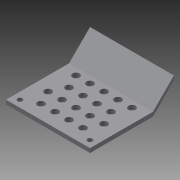
# Autodesk Inventor part: rejilla.ventilador
Saved by Autodesk Inventor 2015 SP1 (Build 190203100, 203)
## iProperties
Created: 2015-07-09
Part Number: rejilla.ventilador
Material: Generic
Document SubType Name: Modeling
Designer: pc
Density: 1 g/cm^3
Appearance: Default
Author: pc
Autodesk Inventor part; units mm, degrees
ref_plane "YZ Plane" through (0, 0, 0) normal (1, 0, 0) x (0, 1, 0)
ref_plane "XZ Plane" through (0, 0, 0) normal (0, 1, 0) x (-1, 0, 0)
ref_plane "XY Plane" through (0, 0, 0) normal (0, 0, 1) x (1, 0, 0)
sketch "Sketch3" plane through (0, 0, 0) normal (1, 0, 0) x (0, 1, 0)
  line L0 (0, 0) -> (45, 0)
  line L1 (45, 0) -> (60, 15)
  line L2 (0, 0) -> (0, 3)
  line L3 (0, 3) -> (45, 3)
  line L4 (45, 3) -> (60, 18)
  line L5 (60, 18) -> (60, 15)
  dimension "d7" = 45
  dimension "d8" = 135
  dimension "d10" = 15
  dimension "d11" = 45
  dimension "d12" = 21.2132
  dimension "d13" = 3
  constraints: 12 end point, 1 coincident, 1 horizontal, 1 parallel, 1 perpendicular, 1 vertical
  measures "d7" distance of L0.start L0.end
  measures "d8" angle of L1 L0
  measures "d10" horizontal distance of L0.end L1.end
  measures "d11" distance of L2.end L3.end
  measures "d12" distance of L3.end L4.end
  measures "d13" distance of L0.start L2.end
extrude "Extrusion3" add sketch "Sketch3" along normal blind 60
sketch "Sketch4" plane through (0, 0, 0) normal (0, 0, -1) x (-1, 0, 0)
  line L0 (0, 0) -> (0, 45) projected
  line L1 (0, 45) -> (-60, 45) projected
  line L2 (-60, 0) -> (-60, 45) projected
  line L3 (0, 0) -> (-60, 0) projected
  circle A0 centre (-55, 5) radius 1.75
  circle A1 centre (-5, 5) radius 1.75
  dimension "d16" = 3.5
  dimension "d18" = 50
  dimension "d19" = 5
  constraints: 2 centre point, 1 equal radius, 1 horizontal alignment
  measures "d16" diameter of A0
  measures "d18" distance of A1.centre A0.centre
  measures "d19" distance from line of L2 A0.centre
extrude "Extrusion4" cut sketch "Sketch4" against normal through all contours A0 | A1
sketch "Sketch5" plane through (0, 0, 3) normal (0, 0, 1) x (1, 0, 0)
  circle A0 centre (55, 5) radius 1.75 projected
  circle A1 centre (5, 5) radius 1.75 projected
  line L0 (0, 45) -> (0, 0) projected
  line L1 (0, 0) -> (60, 0) projected
  line L2 (60, 45) -> (60, 0) projected
  line L3 (0, 45) -> (60, 45) projected
  circle A2 centre (10, 40) radius 2.5
  circle A3 centre (20, 40) radius 2.5
  circle A4 centre (30, 40) radius 2.5
  circle A5 centre (40, 40) radius 2.5
  circle A6 centre (50, 40) radius 2.5
  circle A7 centre (10, 20) radius 2.5
  circle A8 centre (20, 20) radius 2.5
  circle A9 centre (30, 20) radius 2.5
  circle A10 centre (40, 20) radius 2.5
  circle A11 centre (50, 20) radius 2.5
  circle A12 centre (15, 30) radius 2.5
  circle A13 centre (25, 30) radius 2.5
  circle A14 centre (35, 30) radius 2.5
  circle A15 centre (45, 30) radius 2.5
  circle A16 centre (15, 10) radius 2.5
  circle A17 centre (25, 10) radius 2.5
  circle A18 centre (35, 10) radius 2.5
  circle A19 centre (45, 10) radius 2.5
  point P0 (0, 0)
  dimension "d22" = 5
  dimension "d25" = 10
  dimension "d28" = 20
  dimension "d32" = 5
  dimension "d33" = 10
  dimension "d35" = 10
  dimension "d38" = 10
  dimension "d41" = 20
  constraints: 18 centre point, 2 horizontal, 2 vertical, 32 other
  measures "d22" diameter of A2
  measures "d25" distance of A2.centre A3.centre
  measures "d28" distance of A2.centre A7.centre
  measures "d32" diameter of A12
  measures "d33" distance from line of L0 A2.centre
  measures "d35" vertical distance of A12.centre A2.centre
  measures "d38" distance of A12.centre A13.centre
  measures "d41" distance of A12.centre A16.centre
extrude "Extrusion5" cut sketch "Sketch5" against normal through all contours A2 | A3 | A4 | A5 | A6 | A7 | A8 | A9 | A10 | A11 | A12 | A13 | A14 | A15 | A16 | A17 | A18 | A19
body "Solid2"
